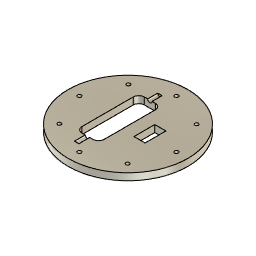
外壳4 v14 (Autodesk Fusion 360 design; units mm, degrees)
Autodesk Fusion 360 part; units mm, degrees
note: some values were not read from the file. Set by a fixed rule: which sketch regions a step uses.
sketch "草图6" plane through (0, 0, 0) normal (0, 0, 1) x (1, 0, 0)
  line L0 (4, 0) -> (12, 0)
  line L1 (16, 4) -> (16, 41)
  line L2 (12, 45) -> (4, 45)
  line L3 (0, 41) -> (0, 4)
  arc A0 (4, 45) -> (0, 41) centre (4, 41) ccw
  arc A1 (16, 41) -> (12, 45) centre (12, 41) ccw
  arc A2 (0, 4) -> (4, 0) centre (4, 4) ccw
  arc A3 (12, 0) -> (16, 4) centre (12, 4) ccw
  line L4 (25, 31.5418) -> (33, 31.5418)
  line L5 (33, 31.5418) -> (33, 16.5418)
  line L6 (33, 16.5418) -> (25, 16.5418)
  line L7 (25, 16.5418) -> (25, 31.5418)
  line L8 (-15, 52.2379) -> (45, 52.2379)
  line L9 (45, 52.2379) -> (45, -7.7621)
  line L10 (45, -7.7621) -> (-15, -7.7621)
  line L11 (-15, -7.7621) -> (-15, 52.2379)
  line L12 (45, -7.7621) -> (-15, 52.2379) construction
  line L13 (-15, -7.7621) -> (45, 52.2379) construction
  circle A4 centre (15, 22.2379) radius 43.1
  point P0 (16, 0)
  point P1 (0, 45)
  dimension "d37" = 4
  dimension "d38" = 4
  dimension "d39" = 4
  dimension "d40" = 4
  dimension "d41" = 45
  dimension "d42" = 16
  dimension "d43" = 8
  dimension "d44" = 15
  dimension "d45" = 60
  dimension "d55" = 60
  dimension "d56" = 86.2
  constraint horizontal L0
  constraint vertical L1
  constraint horizontal L2
  constraint vertical L3
  constraint coincident P1 L2
  constraint coincident P1 L3
  constraint tangent L2 A0
  constraint tangent L3 A0
  constraint tangent L2 A1
  constraint tangent L1 A1
  constraint coincident origin L3
  constraint coincident origin L0
  constraint tangent L3 A2
  constraint tangent L0 A2
  constraint coincident P0 L1
  constraint coincident P0 L0
  constraint tangent L1 A3
  constraint tangent L0 A3
  constraint horizontal L4
  constraint vertical L5
  constraint horizontal L6
  constraint vertical L7
  constraint horizontal L8
  constraint vertical L9
  constraint horizontal L10
  constraint vertical L11
  constraint midpoint L12 A4.centre
  measures "d37" radius of A0
  measures "d38" radius of A1
  measures "d39" radius of A2
  measures "d40" radius of A3
  measures "d41" distance of L0 L2
  measures "d42" distance of L1 L3
  measures "d43" distance of L4.start L4.end
  measures "d44" distance of L4.start L6.end
  measures "d45" distance of L8.start L10.end
  measures "d55" distance of L8.start L8.end
  measures "d56" diameter of A4
extrude "拉伸5" add sketch "草图6" along normal blind 5 contours L8 L9 L10 L11
sketch "草图7" plane through (0, 45, 0) normal (0, -1, 0) x (1, 0, 0)
  line L0 (4, 0) -> (12, 0)
  line L1 (12, 0) -> (12, 5)
  line L2 (12, 5) -> (4, 5)
  line L3 (4, 5) -> (4, 0)
  circle A0 centre (8, 5) radius 1.6
  dimension "d48" = 3.2
  constraint midpoint L2 A0.centre
  measures "d48" diameter of A0
extrude "拉伸6" cut sketch "草图7" along normal blind -10 and the other way blind -55 contours L2 A0 picked at (7.5748, 4.2826)
extrude "拉伸7" add sketch "草图6" along normal blind 5 contours A4
sketch "草图10" plane through (0, 0, 0) normal (0, 0, -1) x (1, 0, 0)
  circle A0 centre (15, -22.2379) radius 43.1
  arc A1 (16, -4) -> (12, 0) centre (12, -4) ccw
  line L0 (16, -4) -> (16, -41)
  arc A2 (12, -45) -> (16, -41) centre (12, -41) ccw
  line L1 (12, -45) -> (4, -45)
  arc A3 (0, -41) -> (4, -45) centre (4, -41) ccw
  line L2 (0, -41) -> (0, -4)
  arc A4 (4, 0) -> (0, -4) centre (4, -4) ccw
  line L3 (4, 0) -> (12, 0)
  line L4 (25, -16.5418) -> (33, -16.5418)
  line L5 (33, -16.5418) -> (33, -31.5418)
  line L6 (33, -31.5418) -> (25, -31.5418)
  line L7 (25, -31.5418) -> (25, -16.5418)
  circle A5 centre (15, -22.2379) radius 35
  circle A6 centre (15, -57.2379) radius 3
  circle A7 centre (15, -57.2379) radius 1.35
  circle A8 centre (50, -22.2379) radius 3
  circle A9 centre (50, -22.2379) radius 1.35
  circle A10 centre (15, 12.7621) radius 3
  circle A11 centre (15, 12.7621) radius 1.35
  circle A12 centre (-20, -22.2379) radius 3
  circle A13 centre (-20, -22.2379) radius 1.35
  line L8 (-7.4138, -45.6983) -> (-7.8923, -46.1073)
  line L9 (-6.756, -46.4514) -> (-7.1427, -46.7964)
  arc A14 (-6.756, -46.4514) -> (-7.4138, -45.6983) centre (-7.0889, -46.0783) ccw
  arc A15 (-7.8923, -46.1073) -> (-7.1427, -46.7964) centre (-8.8265, -47.8757) ccw
  arc A16 (38.8694, -45.1301) -> (39.5585, -44.3806) centre (40.6378, -46.0644) ccw
  line L10 (38.4604, -44.6517) -> (38.8694, -45.1301)
  arc A17 (39.2135, -43.9939) -> (38.4604, -44.6517) centre (38.8404, -44.3268) ccw
  line L11 (39.2135, -43.9939) -> (39.5585, -44.3806)
  arc A18 (37.8923, 1.6315) -> (37.1427, 2.3206) centre (38.8265, 3.3999) ccw
  line L12 (37.4138, 1.2225) -> (37.8923, 1.6315)
  arc A19 (36.756, 1.9756) -> (37.4138, 1.2225) centre (37.0889, 1.6025) ccw
  line L13 (36.756, 1.9756) -> (37.1427, 2.3206)
  arc A20 (-8.8694, 0.6544) -> (-9.5585, -0.0951) centre (-10.6378, 1.5886) ccw
  line L14 (-8.4604, 0.1759) -> (-8.8694, 0.6544)
  arc A21 (-9.2135, -0.4818) -> (-8.4604, 0.1759) centre (-8.8404, -0.149) ccw
  line L15 (-9.2135, -0.4818) -> (-9.5585, -0.0951)
  dimension "d59" = 70
  dimension "d60" = 6
  dimension "d61" = 2.7
  dimension "d63" = 360
  dimension "d68" = 4
  dimension "d69" = 1
  dimension "d71" = 360
  constraint concentric A0 A5
  constraint coincident A5 A6.centre
  constraint concentric A6 A7
  constraint coincident A5 A15.centre
  constraint tangent A14 A15
  constraint tangent L9 A14
  constraint tangent L8 A14
  measures "d59" diameter of A5
  measures "d60" diameter of A6
  measures "d61" diameter of A7
  measures "d68" diameter of A15
  measures "d69" diameter of A14
extrude "拉伸8" cut sketch "草图10" against normal up to surface (5 mm away) contours A5 A9 | A5 A9 | A5 A11 | A5 A11 | A5 A7 | A5 A7 | A5 A13 | A5 A13
extrude "拉伸9" cut sketch "草图10" against normal blind 3 contours A5 A8 A9 | A5 A8 A9 | A5 A10 A11 | A5 A10 A11 | A5 A6 A7 | A5 A6 A7 | A5 A12 A13 | A5 A12 A13
sketch "草图11" plane through (0, 0, 0) normal (0, 0, -1) x (1, 0, 0)
  circle A0 centre (50, -22.2379) radius 3
  circle A1 centre (-20, -22.2379) radius 3
  circle A2 centre (15, -57.2379) radius 3
  circle A3 centre (15, 12.7621) radius 3
  circle A4 centre (15, -22.2379) radius 43.1
  arc A5 (16, -4) -> (12, 0) centre (12, -4) ccw
  line L0 (16, -4) -> (16, -41)
  arc A6 (12, -45) -> (16, -41) centre (12, -41) ccw
  line L1 (12, -45) -> (4, -45)
  arc A7 (0, -41) -> (4, -45) centre (4, -41) ccw
  line L2 (0, -41) -> (0, -4)
  arc A8 (4, 0) -> (0, -4) centre (4, -4) ccw
  line L3 (4, 0) -> (12, 0)
  line L4 (25, -16.5418) -> (33, -16.5418)
  line L5 (33, -16.5418) -> (33, -31.5418)
  line L6 (33, -31.5418) -> (25, -31.5418)
  line L7 (25, -31.5418) -> (25, -16.5418)
  circle A9 centre (15, -22.2379) radius 35
  circle A10 centre (39.6014, 2.6573) radius 1.3
  circle A11 centre (-9.8952, 2.3635) radius 1.3
  circle A12 centre (-9.6014, -47.1331) radius 1.3
  circle A13 centre (39.8952, -46.8393) radius 1.3
  dimension "d74" = 2.6
  dimension "d76" = 360
  constraint concentric A4 A9
  constraint coincident A3.centre A9
  constraint coincident A9 A10.centre
  measures "d74" diameter of A10
extrude "拉伸11" cut sketch "草图11" against normal blind 5 contours A9 A10 | A9 A10 | A9 A13 | A9 A13 | A9 A11 | A9 A11 | A9 A12 | A9 A12
